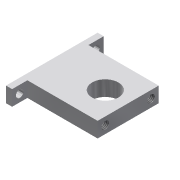
# Autodesk Inventor part: Pipe bracket
Saved by Autodesk Inventor 2014 SP2 (Build 180246200, 246)
## iProperties
Created: 2014-12-08
Part Number: Pipe bracket
Material: Aluminum 6061
Document SubType Name: Modeling
Designer: AlecShufelt
Density: 2.71 g/cm^3
Appearance: Aluminum - Polished
Mass: 95.1834 g
Surface Area: 119.769 cm^2
Volume: 35.123 cm^3
Author: AlecShufelt
Autodesk Inventor part; units mm, degrees
ref_plane "YZ Plane" through (0, 0, 0) normal (1, 0, 0) x (0, 1, 0)
ref_plane "XZ Plane" through (0, 0, 0) normal (0, 1, 0) x (-1, 0, 0)
ref_plane "XY Plane" through (0, 0, 0) normal (0, 0, 1) x (1, 0, 0)
sketch "Sketch1" plane through (0, 0, 0) normal (0, 1, 0) x (-1, 0, 0)
  line L0 (0, 0) -> (63.5, 0)
  line L1 (63.5, 0) -> (63.5, 50.8)
  line L2 (63.5, 50.8) -> (0, 50.8)
  line L3 (0, 50.8) -> (0, 0)
  dimension "d0" = 63.5
  dimension "d1" = 50.8
  constraints: 8 end point, 2 parallel, 1 horizontal, 1 perpendicular
  measures "d0" distance of L2.end L1.end
  measures "d1" distance of L1.end L0.end
extrude "Extrusion1" add sketch "Sketch1" along normal blind 12.7
sketch "Sketch3" plane through (0, 12.7, 0) normal (0, 1, 0) x (1, 0, 0)
  circle A0 centre (-19.05, -25.4) radius 10.9093
  line L0 (-63.5, -50.8) -> (0, -50.8) projected
  line L1 (0, -50.8) -> (0, 0) projected
  dimension "d9" = 21.8186
  dimension "d22" = 19.05
  dimension "d23" = 50.8
  dimension "d24" = 25.4
  constraints: 1 centre point
  measures "d9" diameter of A0
  measures "d22" distance from line of L1 A0.centre
  measures "d23" distance of L0.end L1.end
  measures "d24" distance from line of L0 A0.centre
extrude "Extrusion3" cut sketch "Sketch3" against normal blind 25.4
sketch "Sketch4" plane through (-63.5, 0, 50.8) normal (0, 0, 1) x (1, 0, 0)
  line L0 (0, 12.7) -> (63.5, 12.7) projected
  line L1 (0, 0) -> (0, 12.7) projected
  line L2 (0, 0) -> (5.08, 0)
  line L3 (5.08, 0) -> (5.08, 12.7)
  line L4 (5.08, 12.7) -> (0, 12.7)
  line L5 (0, 12.7) -> (0, 0)
  dimension "d12" = 5.08
  constraints: 8 end point, 2 parallel, 1 horizontal, 1 perpendicular, 1 point on line
  measures "d12" distance of L4.end L3.end
extrude "Extrusion4" add sketch "Sketch4" along normal blind 12.7
sketch "Sketch5" plane through (0, 0, 0) normal (0, 0, -1) x (-1, 0, 0)
  line L0 (0, 12.7) -> (63.5, 12.7) projected
  line L1 (63.5, 0) -> (58.42, 0)
  line L2 (58.42, 0) -> (58.42, 12.7)
  line L3 (58.42, 12.7) -> (63.5, 12.7)
  line L4 (63.5, 12.7) -> (63.5, 0)
  dimension "d15" = 5.08
  constraints: 8 end point, 2 parallel, 1 horizontal, 1 perpendicular, 1 point on line
  measures "d15" distance of L2.end L3.end
extrude "Extrusion5" add sketch "Sketch5" along normal blind 12.7
sketch "Sketch6" plane through (0, 0, 50.8) normal (1, 0, 0) x (0, 0, -1)
  line L0 (50.8, 0) -> (50.8, 12.7) projected
  line L1 (0, 0) -> (0, 12.7) projected
  circle A0 centre (6.35, 6.35) radius 3.175
  circle A1 centre (44.45, 6.35) radius 3.175
  dimension "d18" = 6.35
  dimension "d19" = 6.35
  dimension "d20" = 6.35
  dimension "d21" = 6.35
  constraints: 2 centre point
  measures "d18" diameter of A0
  measures "d19" diameter of A1
  measures "d20" distance from line of L1 A0.centre
  measures "d21" distance from line of L0 A1.centre
extrude "Extrusion6" cut sketch "Sketch6" against normal blind 38.1
thread "Thread1" size "1/4-20 UNC" class "2B" standard "ANSI Unified Screw Threads" full length
thread "Thread2" size "1/4-20 UNC" class "2B" standard "ANSI Unified Screw Threads" full length
sketch "Sketch7" plane through (-58.42, 0, 0) normal (1, 0, 0) x (0, 0, -1)
  circle A0 centre (6.35, 6.35) radius 3.175
  dimension "d31" = 6.35
  constraints: 1 centre point, 1 coincident
  measures "d31" diameter of A0
extrude "Extrusion7" cut sketch "Sketch7" against normal blind 38.1
sketch "Sketch8" plane through (-58.42, 0, 50.8) normal (1, 0, 0) x (0, 0, -1)
  circle A0 centre (-6.35, 6.35) radius 3.175
  point P0 (50.8, 0)
  dimension "d34" = 6.35
  constraints: 1 centre point
  measures "d34" diameter of A0
extrude "Extrusion8" cut sketch "Sketch8" against normal blind 38.1
equation "\"d24\" = 0.5 * d23"
body "Solid1"
